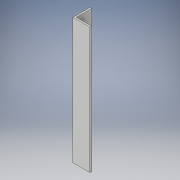
# Autodesk Inventor part: FrameThinBracket
Saved by Autodesk Inventor 2019 (Build 230136000, 136)
## iProperties
Created: 2018-08-17
Part Number: FrameThinBracket
Material: Generic
Document SubType Name: Modeling
Designer: Kitte_X
Density: 1 g/cm^3
Appearance: Default
Author: Kitte_X
Autodesk Inventor part; units mm, degrees
ref_plane "YZ Plane" through (0, 0, 0) normal (1, 0, 0) x (0, 1, 0)
ref_plane "XZ Plane" through (0, 0, 0) normal (0, 1, 0) x (-1, 0, 0)
ref_plane "XY Plane" through (0, 0, 0) normal (0, 0, 1) x (1, 0, 0)
sketch "Sketch1" plane through (0, 0, 0) normal (0, 1, 0) x (-1, 0, 0)
  line L0 (0.8, 8.8) -> (-39.2, 8.8)
  line L1 (-39.2, 8.8) -> (-39.2, 4.8)
  line L2 (-39.2, 4.8) -> (-3.2, 4.8)
  line L3 (-3.2, 4.8) -> (-3.2, -31.2)
  line L4 (-3.2, -31.2) -> (0.8, -31.2)
  line L5 (0.8, -31.2) -> (0.8, 8.8)
  point P0 (0, 0)
  dimension "d0" = 4
  dimension "d1" = 4
  dimension "d2" = 40
  dimension "d3" = 40
  constraints: 12 end point, 4 perpendicular, 1 horizontal, 1 parallel
  measures "d0" distance between parallel lines of L5 L3
  measures "d1" distance between parallel lines of L0 L2
  measures "d2" distance of L0.start L0.end
  measures "d3" distance of L4.end L0.start
extrude "Extrusion1" add sketch "Sketch1" along normal blind 294
body "Solid1"
